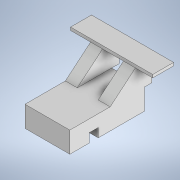
# Autodesk Inventor part: FP Rear Hood
Saved by Autodesk Inventor 2020 (Build 240168000, 168)
## iProperties
Created: 2021-04-14
Part Number: FP Rear Hood
Material: Generic
Document SubType Name: Modeling
Designer: austi
Density: 1 g/cm^3
Appearance: Default
Author: austi
Autodesk Inventor part; units mm, degrees
ref_plane "YZ Plane" through (0, 0, 0) normal (1, 0, 0) x (0, 1, 0)
ref_plane "XZ Plane" through (0, 0, 0) normal (0, 1, 0) x (-1, 0, 0)
ref_plane "XY Plane" through (0, 0, 0) normal (0, 0, 1) x (1, 0, 0)
sketch "Sketch1" plane through (0, 0, 0) normal (0, 1, 0) x (-1, 0, 0)
  line L0 (9.8, 0) -> (-9.8, 0) projected
  line L1 (0, -35) -> (0, 35) projected
  line L2 (7, 25) -> (-7, 25)
  line L3 (-7, -25) -> (7, -25)
  line L4 (7, -25) -> (7, 25)
  line L5 (-7, 12) -> (-1, 12)
  line L6 (-1, 12) -> (-1, 6)
  line L7 (-1, 6) -> (-7, 6)
  line L8 (-7, 25) -> (-7, 12)
  line L9 (-7, 6) -> (-7, -25)
  point P0 (0, 0)
  point P1 (7, 0)
  point P2 (0, 25)
  dimension "d0" = 14
  dimension "d1" = 50
  dimension "d2" = 6
  dimension "d3" = 6
  dimension "d4" = 13
  constraints: 16 end point, 5 perpendicular, 4 parallel, 2 horizontal, 2 midpoint, 1 horizontal alignment, 1 vertical alignment, 1 other
  measures "d0" distance of L3.end L3.start
  measures "d1" distance of L3.start L2.end
  measures "d2" distance of L5.start L5.end
  measures "d3" distance of L5.end L6.end
  measures "d4" distance of L5.start L2.end
extrude "Extrusion1" add sketch "Sketch1" along normal blind 30
sketch "Sketch2" plane through (-7, 0, -25) normal (-1, 0, 0) x (0, 0, 1)
  line L0 (23, 0) -> (23, 8)
  line L1 (23, 0) -> (-5, 0)
  line L2 (0, 0) -> (50, 0) projected
  line L3 (-5, 0) -> (-5, 8)
  line L4 (-5, 8) -> (23, 8)
  line L5 (-5, 22) -> (23, 22)
  line L6 (23, 22) -> (23, 30)
  line L7 (23, 30) -> (-5, 30)
  line L8 (-5, 30) -> (-5, 22)
  line L9 (0, 30) -> (50, 30) projected
  line L10 (5, 0) -> (5, 8)
  line L11 (5, 22) -> (5, 30)
  point P0 (25, 0)
  point P1 (5, 0)
  dimension "d8" = 8
  dimension "d9" = 23
  dimension "d10" = 28
  dimension "d11" = 28
  dimension "d12" = 8
  dimension "d14" = 10
  constraints: 20 end point, 6 point on line, 4 perpendicular, 2 parallel, 2 vertical, 2 vertical alignment, 1 collinear, 1 horizontal
  measures "d8" distance of L0.start L0.end
  measures "d9" distance from line of L0 L2.start
  measures "d10" distance of L0.start L1.end
  measures "d11" distance of L7.end L6.end
  measures "d12" distance of L6.end L5.end
  measures "d14" distance of L10.end L3.end
extrude "Extrusion2" add sketch "Sketch2" along normal blind 15 contours L1 L3 L4 L10 | L8 L7 L11 L5
sketch "Sketch3" plane through (0, 30, 0) normal (0, 1, 0) x (1, 0, 0)
  line L0 (-7, 20) -> (-7, -25) projected
  line L1 (-7, 20) -> (-22, 20) projected
  line L2 (-22, 20) -> (-22, 30) projected
  line L3 (-7, 20) -> (-7, 2)
  line L4 (-7, 20) -> (-22, 20) projected
  line L5 (-7, 2) -> (-22, 20)
  line L6 (-22, 20) -> (-7, 20)
  point P0 (0, 0)
  dimension "d17" = 18
  constraints: 6 end point, 1 collinear, 1 point on line
  measures "d17" distance of L0.start L3.end
extrude "Extrusion3" add sketch "Sketch3" against normal blind 8
sketch "Sketch4" plane through (0, 0, 0) normal (0, -1, 0) x (1, 0, 0)
  line L0 (-7, -20) -> (-7, 25) projected
  line L1 (-7, -20) -> (-7, -2)
  line L2 (-22, -20) -> (-22, -30) projected
  line L3 (-7, -2) -> (-22, -20)
  line L4 (-22, -20) -> (-7, -20)
  point P0 (0, 0)
  dimension "d20" = 18
  constraints: 6 end point, 1 perpendicular, 1 point on line
  measures "d20" distance of L0.start L1.end
extrude "Extrusion4" add sketch "Sketch4" against normal blind 8
sketch "Sketch5" plane through (-22, 0, -25) normal (-1, 0, 0) x (0, 0, 1)
  line L0 (-5, 0) -> (5, 0) projected
  line L1 (-5, 8) -> (-5, 0) projected
  line L2 (5, 8) -> (-5, 8) projected
  line L3 (5, 0) -> (5, 8) projected
  line L4 (5, 22) -> (5, 30) projected
  line L5 (-5, 22) -> (5, 22) projected
  line L6 (-5, 30) -> (-5, 22) projected
  line L7 (5, 30) -> (-5, 30) projected
  line L8 (-7, -12.5) -> (7, -12.5)
  line L9 (7, -12.5) -> (7, 42.5)
  line L10 (7, 42.5) -> (-7, 42.5)
  line L11 (-7, 42.5) -> (-7, -12.5)
  line L12 (0, 8) -> (0, 22) projected
  point P0 (25, 0)
  point P1 (0, -12.5)
  point P2 (0, 0)
  point P3 (-7, 15)
  point P4 (0, 15)
  dimension "d23" = 14
  dimension "d24" = 55
  constraints: 8 end point, 4 midpoint, 2 parallel, 1 horizontal, 1 horizontal alignment, 1 perpendicular, 1 vertical alignment
  measures "d23" distance of L10.end L9.end
  measures "d24" distance of L9.end L8.end
extrude "Extrusion5" add sketch "Sketch5" along normal blind 2 contours L1 L2 L3 L0 | L5 L6 L7 L4 | L11 L10 L9 L8
body "Solid1"
